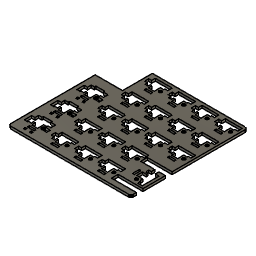
bottomplate (Autodesk Fusion 360 design; units mm, degrees)
Autodesk Fusion 360 part; units mm, degrees
(part 1 of 5)
sketch "スケッチ1" plane through (0, 0, 0) normal (0, 0, 1) x (1, 0, 0)
  line L0 (62.5173, -152.0791) -> (62.5309, -152.0926)
  line L1 (62.5309, -152.0926) -> (62.5328, -152.1022)
  line L2 (62.5328, -152.1022) -> (62.5328, -153.5905)
  line L3 (62.5328, -153.5905) -> (62.5309, -153.6001)
  line L4 (62.5309, -153.6001) -> (62.5173, -153.6136)
  line L5 (62.5173, -153.6136) -> (62.5078, -153.6155)
  line L6 (62.5078, -153.6155) -> (61.0195, -153.6155)
  line L7 (61.0195, -153.6155) -> (61.0099, -153.6136)
  line L8 (61.0099, -153.6136) -> (60.9964, -153.6001)
  line L9 (60.9964, -153.6001) -> (60.9945, -153.5905)
  line L10 (60.9945, -153.5905) -> (60.9945, -152.1022)
  line L11 (60.9945, -152.1022) -> (60.9964, -152.0926)
  line L12 (60.9964, -152.0926) -> (61.0099, -152.0791)
  line L13 (61.0099, -152.0791) -> (61.0195, -152.0772)
  line L14 (61.0195, -152.0772) -> (62.5078, -152.0772)
  line L15 (62.5078, -152.0772) -> (62.5173, -152.0791)
  line L16 (61.0445, -152.1272) -> (61.0445, -153.5655)
  line L17 (61.0445, -153.5655) -> (62.4828, -153.5655)
  line L18 (62.4828, -153.5655) -> (62.4828, -152.1272)
  line L19 (62.4828, -152.1272) -> (61.0445, -152.1272)
  line L20 (67.5775, -152.0791) -> (67.591, -152.0926)
  line L21 (67.591, -152.0926) -> (67.5929, -152.1022)
  line L22 (67.5929, -152.1022) -> (67.5929, -153.5905)
  line L23 (67.5929, -153.5905) -> (67.591, -153.6001)
  line L24 (67.591, -153.6001) -> (67.5775, -153.6136)
  line L25 (67.5775, -153.6136) -> (67.5679, -153.6155)
  line L26 (67.5679, -153.6155) -> (66.0796, -153.6155)
  line L27 (66.0796, -153.6155) -> (66.0701, -153.6136)
  line L28 (66.0701, -153.6136) -> (66.0565, -153.6001)
  line L29 (66.0565, -153.6001) -> (66.0546, -153.5905)
  line L30 (66.0546, -153.5905) -> (66.0546, -152.1022)
  line L31 (66.0546, -152.1022) -> (66.0565, -152.0926)
  line L32 (66.0565, -152.0926) -> (66.0701, -152.0791)
  line L33 (66.0701, -152.0791) -> (66.0796, -152.0772)
  line L34 (66.0796, -152.0772) -> (67.5679, -152.0772)
  line L35 (67.5679, -152.0772) -> (67.5775, -152.0791)
  line L36 (66.1046, -152.1272) -> (66.1046, -153.5655)
  line L37 (66.1046, -153.5655) -> (67.5429, -153.5655)
  line L38 (67.5429, -153.5655) -> (67.5429, -152.1272)
  line L39 (67.5429, -152.1272) -> (66.1046, -152.1272)
  line L40 (88.4346, -151.6269) -> (88.4481, -151.6404)
  line L41 (88.4481, -151.6404) -> (88.45, -151.65)
  line L42 (88.45, -151.65) -> (88.45, -153.15)
  line L43 (88.45, -153.15) -> (88.4481, -153.1596)
  line L44 (88.4481, -153.1596) -> (88.4346, -153.1731)
  line L45 (88.4346, -153.1731) -> (88.425, -153.175)
  line L46 (88.425, -153.175) -> (83.025, -153.175)
  line L47 (83.025, -153.175) -> (83.0154, -153.1731)
  line L48 (83.0154, -153.1731) -> (83.0019, -153.1596)
  line L49 (83.0019, -153.1596) -> (83, -153.15)
  line L50 (83, -153.15) -> (83, -151.65)
  line L51 (83, -151.65) -> (83.0019, -151.6404)
  line L52 (83.0019, -151.6404) -> (83.0154, -151.6269)
  line L53 (83.0154, -151.6269) -> (83.025, -151.625)
  line L54 (83.025, -151.625) -> (88.425, -151.625)
  line L55 (88.425, -151.625) -> (88.4346, -151.6269)
  line L56 (83.05, -151.675) -> (83.05, -153.125)
  line L57 (83.05, -153.125) -> (88.4, -153.125)
  line L58 (88.4, -153.125) -> (88.4, -151.675)
  line L59 (88.4, -151.675) -> (83.05, -151.675)
  line L60 (107.4846, -151.6269) -> (107.4981, -151.6404)
  line L61 (107.4981, -151.6404) -> (107.5, -151.65)
  line L62 (107.5, -151.65) -> (107.5, -153.15)
  line L63 (107.5, -153.15) -> (107.4981, -153.1596)
  line L64 (107.4981, -153.1596) -> (107.4846, -153.1731)
  line L65 (107.4846, -153.1731) -> (107.475, -153.175)
  line L66 (107.475, -153.175) -> (102.075, -153.175)
  line L67 (102.075, -153.175) -> (102.0654, -153.1731)
  line L68 (102.0654, -153.1731) -> (102.0519, -153.1596)
  line L69 (102.0519, -153.1596) -> (102.05, -153.15)
  line L70 (102.05, -153.15) -> (102.05, -151.65)
  line L71 (102.05, -151.65) -> (102.0519, -151.6404)
  line L72 (102.0519, -151.6404) -> (102.0654, -151.6269)
  line L73 (102.0654, -151.6269) -> (102.075, -151.625)
  line L74 (102.075, -151.625) -> (107.475, -151.625)
  line L75 (107.475, -151.625) -> (107.4846, -151.6269)
  line L76 (102.1, -151.675) -> (102.1, -153.125)
  line L77 (102.1, -153.125) -> (107.45, -153.125)
  line L78 (107.45, -153.125) -> (107.45, -151.675)
  line L79 (107.45, -151.675) -> (102.1, -151.675)
  line L80 (126.5346, -151.6269) -> (126.5481, -151.6404)
  line L81 (126.5481, -151.6404) -> (126.55, -151.65)
  line L82 (126.55, -151.65) -> (126.55, -153.15)
  line L83 (126.55, -153.15) -> (126.5481, -153.1596)
  line L84 (126.5481, -153.1596) -> (126.5346, -153.1731)
  line L85 (126.5346, -153.1731) -> (126.525, -153.175)
  line L86 (126.525, -153.175) -> (121.125, -153.175)
  line L87 (121.125, -153.175) -> (121.1154, -153.1731)
  line L88 (121.1154, -153.1731) -> (121.1019, -153.1596)
  line L89 (121.1019, -153.1596) -> (121.1, -153.15)
  line L90 (121.1, -153.15) -> (121.1, -151.65)
  line L91 (121.1, -151.65) -> (121.1019, -151.6404)
  line L92 (121.1019, -151.6404) -> (121.1154, -151.6269)
  line L93 (121.1154, -151.6269) -> (121.125, -151.625)
  line L94 (121.125, -151.625) -> (126.525, -151.625)
  line L95 (126.525, -151.625) -> (126.5346, -151.6269)
  line L96 (121.15, -151.675) -> (121.15, -153.125)
  line L97 (121.15, -153.125) -> (126.5, -153.125)
  line L98 (126.5, -153.125) -> (126.5, -151.675)
  line L99 (126.5, -151.675) -> (121.15, -151.675)
  line L100 (67.0033, -149.2457) -> (67.0168, -149.2592)
  line L101 (67.0168, -149.2592) -> (67.0187, -149.2687)
  line L102 (67.0187, -149.2687) -> (67.0187, -150.7687)
  line L103 (67.0187, -150.7687) -> (67.0168, -150.7783)
  line L104 (67.0168, -150.7783) -> (67.0033, -150.7918)
  line L105 (67.0033, -150.7918) -> (66.9938, -150.7937)
  line L106 (66.9938, -150.7937) -> (61.5938, -150.7937)
  line L107 (61.5938, -150.7937) -> (61.5842, -150.7918)
  line L108 (61.5842, -150.7918) -> (61.5707, -150.7783)
  line L109 (61.5707, -150.7783) -> (61.5688, -150.7687)
  line L110 (61.5688, -150.7687) -> (61.5688, -149.2687)
  line L111 (61.5688, -149.2687) -> (61.5707, -149.2592)
  line L112 (61.5707, -149.2592) -> (61.5842, -149.2457)
  line L113 (61.5842, -149.2457) -> (61.5938, -149.2438)
  line L114 (61.5938, -149.2438) -> (66.9938, -149.2438)
  line L115 (66.9938, -149.2438) -> (67.0033, -149.2457)
  line L116 (61.6188, -149.2937) -> (61.6188, -150.7438)
  line L117 (61.6188, -150.7438) -> (66.9688, -150.7438)
  line L118 (66.9688, -150.7438) -> (66.9688, -149.2937)
  line L119 (66.9688, -149.2937) -> (61.6187, -149.2937)
  line L120 (93.1758, -140.4705) -> (93.1894, -140.4841)
  line L121 (93.1894, -140.4841) -> (93.1913, -140.4936)
  line L122 (93.1913, -140.4936) -> (93.1913, -144.0655)
  line L123 (93.1913, -144.0655) -> (93.1894, -144.0751)
  line L124 (93.1894, -144.0751) -> (93.1758, -144.0886)
  line L125 (93.1758, -144.0886) -> (93.1663, -144.0905)
  line L126 (93.1663, -144.0905) -> (90.81, -144.0905)
  line L127 (90.81, -144.0905) -> (90.81, -144.9585)
  line L128 (90.81, -144.9585) -> (90.8081, -144.968)
  line L129 (90.8081, -144.968) -> (90.7946, -144.9816)
  line L130 (90.7946, -144.9816) -> (90.785, -144.9835)
  line L131 (90.785, -144.9835) -> (88.1311, -144.9835)
  line L132 (88.1311, -144.9835) -> (88.1311, -148.828)
  line L133 (88.1311, -148.828) -> (88.1311, -150.0186)
  line L134 (88.1311, -150.0186) -> (88.1292, -150.0282)
  line L135 (88.1292, -150.0282) -> (88.1157, -150.0417)
  line L136 (88.1157, -150.0417) -> (88.1061, -150.0436)
  line L137 (88.1061, -150.0436) -> (83.6413, -150.0436)
  line L138 (83.6413, -150.0436) -> (83.3436, -150.0436)
  line L139 (83.3436, -150.0436) -> (83.334, -150.0417)
  line L140 (83.334, -150.0417) -> (83.3205, -150.0282)
  line L141 (83.3205, -150.0282) -> (83.3186, -150.0186)
  line L142 (83.3186, -150.0186) -> (83.3186, -147.0671)
  line L143 (83.3186, -147.0671) -> (81.8803, -147.0671)
  line L144 (81.8803, -147.0671) -> (81.8803, -148.828)
  line L145 (81.8803, -148.828) -> (81.8784, -148.8376)
  line L146 (81.8784, -148.8376) -> (81.8649, -148.8511)
  line L147 (81.8649, -148.8511) -> (81.8553, -148.853)
  line L148 (81.8553, -148.853) -> (79.4741, -148.853)
  line L149 (79.4741, -148.853) -> (79.4645, -148.8511)
  line L150 (79.4645, -148.8511) -> (79.451, -148.8376)
  line L151 (79.451, -148.8376) -> (79.4491, -148.828)
  line L152 (79.4491, -148.828) -> (79.4491, -146.7694)
  line L153 (79.4491, -146.7694) -> (77.0928, -146.7694)
  line L154 (77.0928, -146.7694) -> (77.0833, -146.7675)
  line L155 (77.0833, -146.7675) -> (77.0697, -146.754)
  line L156 (77.0697, -146.754) -> (77.0678, -146.7444)
  line L157 (77.0678, -146.7444) -> (77.0678, -143.4702)
  line L158 (77.0678, -143.4702) -> (77.0697, -143.4606)
  line L159 (77.0697, -143.4606) -> (77.0833, -143.4471)
  line L160 (77.0833, -143.4471) -> (77.0928, -143.4452)
  line L161 (77.0928, -143.4452) -> (79.4491, -143.4452)
  line L162 (79.4491, -143.4452) -> (79.4491, -140.4936)
  line L163 (79.4491, -140.4936) -> (79.451, -140.4841)
  line L164 (79.451, -140.4841) -> (79.4645, -140.4705)
  line L165 (79.4645, -140.4705) -> (79.4741, -140.4686)
  line L166 (79.4741, -140.4686) -> (93.1663, -140.4686)
  line L167 (93.1663, -140.4686) -> (93.1758, -140.4705)
  line L168 (79.4991, -140.5186) -> (79.4991, -143.4702)
  line L169 (79.4991, -143.4702) -> (79.4972, -143.4798)
  line L170 (79.4972, -143.4798) -> (79.4836, -143.4933)
  line L171 (79.4836, -143.4933) -> (79.4741, -143.4952)
  line L172 (79.4741, -143.4952) -> (77.1178, -143.4952)
  line L173 (77.1178, -143.4952) -> (77.1178, -146.7194)
  line L174 (77.1178, -146.7194) -> (79.4741, -146.7194)
  line L175 (79.4741, -146.7194) -> (79.4836, -146.7213)
  line L176 (79.4836, -146.7213) -> (79.4972, -146.7348)
  line L177 (79.4972, -146.7348) -> (79.4991, -146.7444)
  line L178 (79.4991, -146.7444) -> (79.4991, -148.803)
  line L179 (79.4991, -148.803) -> (81.8303, -148.803)
  line L180 (81.8303, -148.803) -> (81.8303, -147.0421)
  line L181 (81.8303, -147.0421) -> (81.8322, -147.0325)
  line L182 (81.8322, -147.0325) -> (81.8458, -147.019)
  line L183 (81.8458, -147.019) -> (81.8553, -147.0171)
  line L184 (81.8553, -147.0171) -> (83.3436, -147.0171)
  line L185 (83.3436, -147.0171) -> (83.3532, -147.019)
  line L186 (83.3532, -147.019) -> (83.3667, -147.0325)
  line L187 (83.3667, -147.0325) -> (83.3686, -147.0421)
  line L188 (83.3686, -147.0421) -> (83.3686, -149.9936)
  line L189 (83.3686, -149.9936) -> (83.6413, -149.9936)
  line L190 (83.6413, -149.9936) -> (88.0811, -149.9936)
  line L191 (88.0811, -149.9936) -> (88.0811, -148.828)
  line L192 (88.0811, -148.828) -> (88.0811, -144.9585)
  line L193 (88.0811, -144.9585) -> (88.083, -144.9489)
  line L194 (88.083, -144.9489) -> (88.0965, -144.9354)
  line L195 (88.0965, -144.9354) -> (88.1061, -144.9335)
  line L196 (88.1061, -144.9335) -> (90.76, -144.9335)
  line L197 (90.76, -144.9335) -> (90.76, -144.0655)
  line L198 (90.76, -144.0655) -> (90.7619, -144.0559)
  line L199 (90.7619, -144.0559) -> (90.7754, -144.0424)
  line L200 (90.7754, -144.0424) -> (90.785, -144.0405)
  line L201 (90.785, -144.0405) -> (93.1413, -144.0405)
  line L202 (93.1413, -144.0405) -> (93.1413, -140.5186)
  line L203 (93.1413, -140.5186) -> (79.4991, -140.5186)
  line L204 (112.2258, -140.4705) -> (112.2394, -140.4841)
  line L205 (112.2394, -140.4841) -> (112.2413, -140.4936)
  line L206 (112.2413, -140.4936) -> (112.2413, -144.0655)
  line L207 (112.2413, -144.0655) -> (112.2394, -144.0751)
  line L208 (112.2394, -144.0751) -> (112.2258, -144.0886)
  line L209 (112.2258, -144.0886) -> (112.2163, -144.0905)
  line L210 (112.2163, -144.0905) -> (109.86, -144.0905)
  line L211 (109.86, -144.0905) -> (109.86, -144.9585)
  line L212 (109.86, -144.9585) -> (109.8581, -144.968)
  line L213 (109.8581, -144.968) -> (109.8446, -144.9816)
  line L214 (109.8446, -144.9816) -> (109.835, -144.9835)
  line L215 (109.835, -144.9835) -> (107.1811, -144.9835)
  line L216 (107.1811, -144.9835) -> (107.1811, -148.828)
  line L217 (107.1811, -148.828) -> (107.1811, -150.0186)
  line L218 (107.1811, -150.0186) -> (107.1792, -150.0282)
  line L219 (107.1792, -150.0282) -> (107.1657, -150.0417)
  line L220 (107.1657, -150.0417) -> (107.1561, -150.0436)
  line L221 (107.1561, -150.0436) -> (102.6913, -150.0436)
  line L222 (102.6913, -150.0436) -> (102.3936, -150.0436)
  line L223 (102.3936, -150.0436) -> (102.384, -150.0417)
  line L224 (102.384, -150.0417) -> (102.3705, -150.0282)
  line L225 (102.3705, -150.0282) -> (102.3686, -150.0186)
  line L226 (102.3686, -150.0186) -> (102.3686, -147.0671)
  line L227 (102.3686, -147.0671) -> (100.9303, -147.0671)
  line L228 (100.9303, -147.0671) -> (100.9303, -148.828)
  line L229 (100.9303, -148.828) -> (100.9284, -148.8376)
  line L230 (100.9284, -148.8376) -> (100.9149, -148.8511)
  line L231 (100.9149, -148.8511) -> (100.9053, -148.853)
  line L232 (100.9053, -148.853) -> (98.5241, -148.853)
  line L233 (98.5241, -148.853) -> (98.5145, -148.8511)
  line L234 (98.5145, -148.8511) -> (98.501, -148.8376)
  line L235 (98.501, -148.8376) -> (98.4991, -148.828)
  line L236 (98.4991, -148.828) -> (98.4991, -146.7694)
  line L237 (98.4991, -146.7694) -> (96.1428, -146.7694)
  line L238 (96.1428, -146.7694) -> (96.1333, -146.7675)
  line L239 (96.1333, -146.7675) -> (96.1197, -146.754)
  line L240 (96.1197, -146.754) -> (96.1178, -146.7444)
  line L241 (96.1178, -146.7444) -> (96.1178, -143.4702)
  line L242 (96.1178, -143.4702) -> (96.1197, -143.4606)
  line L243 (96.1197, -143.4606) -> (96.1333, -143.4471)
  line L244 (96.1333, -143.4471) -> (96.1428, -143.4452)
  line L245 (96.1428, -143.4452) -> (98.4991, -143.4452)
  line L246 (98.4991, -143.4452) -> (98.4991, -140.4936)
  line L247 (98.4991, -140.4936) -> (98.501, -140.4841)
  line L248 (98.501, -140.4841) -> (98.5145, -140.4705)
  line L249 (98.5145, -140.4705) -> (98.5241, -140.4686)
  line L250 (98.5241, -140.4686) -> (112.2163, -140.4686)
  line L251 (112.2163, -140.4686) -> (112.2258, -140.4705)
  line L252 (98.5491, -140.5186) -> (98.5491, -143.4702)
  line L253 (98.5491, -143.4702) -> (98.5472, -143.4798)
  line L254 (98.5472, -143.4798) -> (98.5336, -143.4933)
  line L255 (98.5336, -143.4933) -> (98.5241, -143.4952)
  line L256 (98.5241, -143.4952) -> (96.1678, -143.4952)
  line L257 (96.1678, -143.4952) -> (96.1678, -146.7194)
  line L258 (96.1678, -146.7194) -> (98.5241, -146.7194)
  line L259 (98.5241, -146.7194) -> (98.5336, -146.7213)
  line L260 (98.5336, -146.7213) -> (98.5472, -146.7348)
  line L261 (98.5472, -146.7348) -> (98.5491, -146.7444)
  line L262 (98.5491, -146.7444) -> (98.5491, -148.803)
  line L263 (98.5491, -148.803) -> (100.8803, -148.803)
  line L264 (100.8803, -148.803) -> (100.8803, -147.0421)
  line L265 (100.8803, -147.0421) -> (100.8822, -147.0325)
  line L266 (100.8822, -147.0325) -> (100.8958, -147.019)
  line L267 (100.8958, -147.019) -> (100.9053, -147.0171)
  line L268 (100.9053, -147.0171) -> (102.3936, -147.0171)
  line L269 (102.3936, -147.0171) -> (102.4032, -147.019)
  line L270 (102.4032, -147.019) -> (102.4167, -147.0325)
  line L271 (102.4167, -147.0325) -> (102.4186, -147.0421)
  line L272 (102.4186, -147.0421) -> (102.4186, -149.9936)
  line L273 (102.4186, -149.9936) -> (102.6913, -149.9936)
  line L274 (102.6913, -149.9936) -> (107.1311, -149.9936)
  line L275 (107.1311, -149.9936) -> (107.1311, -148.828)
  line L276 (107.1311, -148.828) -> (107.1311, -144.9585)
  line L277 (107.1311, -144.9585) -> (107.133, -144.9489)
  line L278 (107.133, -144.9489) -> (107.1465, -144.9354)
  line L279 (107.1465, -144.9354) -> (107.1561, -144.9335)
  line L280 (107.1561, -144.9335) -> (109.81, -144.9335)
  line L281 (109.81, -144.9335) -> (109.81, -144.0655)
  line L282 (109.81, -144.0655) -> (109.8119, -144.0559)
  line L283 (109.8119, -144.0559) -> (109.8254, -144.0424)
  line L284 (109.8254, -144.0424) -> (109.835, -144.0405)
  line L285 (109.835, -144.0405) -> (112.1913, -144.0405)
  line L286 (112.1913, -144.0405) -> (112.1913, -140.5186)
  line L287 (112.1913, -140.5186) -> (98.5491, -140.5186)
  line L288 (131.2758, -140.4705) -> (131.2894, -140.4841)
  line L289 (131.2894, -140.4841) -> (131.2913, -140.4936)
  line L290 (131.2913, -140.4936) -> (131.2913, -144.0655)
  line L291 (131.2913, -144.0655) -> (131.2894, -144.0751)
  line L292 (131.2894, -144.0751) -> (131.2758, -144.0886)
  line L293 (131.2758, -144.0886) -> (131.2663, -144.0905)
  line L294 (131.2663, -144.0905) -> (128.91, -144.0905)
  line L295 (128.91, -144.0905) -> (128.91, -144.9585)
  line L296 (128.91, -144.9585) -> (128.9081, -144.968)
  line L297 (128.9081, -144.968) -> (128.8946, -144.9816)
  line L298 (128.8946, -144.9816) -> (128.885, -144.9835)
  line L299 (128.885, -144.9835) -> (126.2311, -144.9835)
  line L300 (126.2311, -144.9835) -> (126.2311, -148.828)
  line L301 (126.2311, -148.828) -> (126.2311, -150.0186)
  line L302 (126.2311, -150.0186) -> (126.2292, -150.0282)
  line L303 (126.2292, -150.0282) -> (126.2157, -150.0417)
  line L304 (126.2157, -150.0417) -> (126.2061, -150.0436)
  line L305 (126.2061, -150.0436) -> (121.7413, -150.0436)
  line L306 (121.7413, -150.0436) -> (121.4436, -150.0436)
  line L307 (121.4436, -150.0436) -> (121.434, -150.0417)
  line L308 (121.434, -150.0417) -> (121.4205, -150.0282)
  line L309 (121.4205, -150.0282) -> (121.4186, -150.0186)
  line L310 (121.4186, -150.0186) -> (121.4186, -147.0671)
  line L311 (121.4186, -147.0671) -> (119.9803, -147.0671)
  line L312 (119.9803, -147.0671) -> (119.9803, -148.828)
  line L313 (119.9803, -148.828) -> (119.9784, -148.8376)
  line L314 (119.9784, -148.8376) -> (119.9649, -148.8511)
  line L315 (119.9649, -148.8511) -> (119.9553, -148.853)
  line L316 (119.9553, -148.853) -> (117.5741, -148.853)
  line L317 (117.5741, -148.853) -> (117.5645, -148.8511)
  line L318 (117.5645, -148.8511) -> (117.551, -148.8376)
  line L319 (117.551, -148.8376) -> (117.5491, -148.828)
  line L320 (117.5491, -148.828) -> (117.5491, -146.7694)
  line L321 (117.5491, -146.7694) -> (115.1928, -146.7694)
  line L322 (115.1928, -146.7694) -> (115.1833, -146.7675)
  line L323 (115.1833, -146.7675) -> (115.1697, -146.754)
  line L324 (115.1697, -146.754) -> (115.1678, -146.7444)
  line L325 (115.1678, -146.7444) -> (115.1678, -143.4702)
  line L326 (115.1678, -143.4702) -> (115.1697, -143.4606)
  line L327 (115.1697, -143.4606) -> (115.1833, -143.4471)
  line L328 (115.1833, -143.4471) -> (115.1928, -143.4452)
  line L329 (115.1928, -143.4452) -> (117.5491, -143.4452)
  line L330 (117.5491, -143.4452) -> (117.5491, -140.4936)
  line L331 (117.5491, -140.4936) -> (117.551, -140.4841)
  line L332 (117.551, -140.4841) -> (117.5645, -140.4705)
  line L333 (117.5645, -140.4705) -> (117.5741, -140.4686)
  line L334 (117.5741, -140.4686) -> (131.2663, -140.4686)
  line L335 (131.2663, -140.4686) -> (131.2758, -140.4705)
  line L336 (117.5991, -140.5186) -> (117.5991, -143.4702)
  line L337 (117.5991, -143.4702) -> (117.5972, -143.4798)
  line L338 (117.5972, -143.4798) -> (117.5836, -143.4933)
  line L339 (117.5836, -143.4933) -> (117.5741, -143.4952)
  line L340 (117.5741, -143.4952) -> (115.2178, -143.4952)
  line L341 (115.2178, -143.4952) -> (115.2178, -146.7194)
  line L342 (115.2178, -146.7194) -> (117.5741, -146.7194)
  line L343 (117.5741, -146.7194) -> (117.5836, -146.7213)
  line L344 (117.5836, -146.7213) -> (117.5972, -146.7348)
  line L345 (117.5972, -146.7348) -> (117.5991, -146.7444)
  line L346 (117.5991, -146.7444) -> (117.5991, -148.803)
  line L347 (117.5991, -148.803) -> (119.9303, -148.803)
  line L348 (119.9303, -148.803) -> (119.9303, -147.0421)
  line L349 (119.9303, -147.0421) -> (119.9322, -147.0325)
  line L350 (119.9322, -147.0325) -> (119.9458, -147.019)
  line L351 (119.9458, -147.019) -> (119.9553, -147.0171)
  line L352 (119.9553, -147.0171) -> (121.4436, -147.0171)
  line L353 (121.4436, -147.0171) -> (121.4532, -147.019)
  line L354 (121.4532, -147.019) -> (121.4667, -147.0325)
  line L355 (121.4667, -147.0325) -> (121.4686, -147.0421)
  line L356 (121.4686, -147.0421) -> (121.4686, -149.9936)
  line L357 (121.4686, -149.9936) -> (121.7413, -149.9936)
  line L358 (121.7413, -149.9936) -> (126.1811, -149.9936)
  line L359 (126.1811, -149.9936) -> (126.1811, -148.828)
  line L360 (126.1811, -148.828) -> (126.1811, -144.9585)
  line L361 (126.1811, -144.9585) -> (126.183, -144.9489)
  line L362 (126.183, -144.9489) -> (126.1965, -144.9354)
  line L363 (126.1965, -144.9354) -> (126.2061, -144.9335)
  line L364 (126.2061, -144.9335) -> (128.86, -144.9335)
  line L365 (128.86, -144.9335) -> (128.86, -144.0655)
  line L366 (128.86, -144.0655) -> (128.8619, -144.0559)
  line L367 (128.8619, -144.0559) -> (128.8754, -144.0424)
  line L368 (128.8754, -144.0424) -> (128.885, -144.0405)
  line L369 (128.885, -144.0405) -> (131.2413, -144.0405)
  line L370 (131.2413, -144.0405) -> (131.2413, -140.5186)
  line L371 (131.2413, -140.5186) -> (117.5991, -140.5186)
  line L372 (90.9961, -146.4402) -> (91.2008, -146.4951)
  line L373 (91.2008, -146.4951) -> (91.3928, -146.5846)
  line L374 (91.3928, -146.5846) -> (91.5664, -146.7062)
  line L375 (91.5664, -146.7062) -> (91.7162, -146.856)
  line L376 (91.7162, -146.856) -> (91.8378, -147.0296)
  line L377 (91.8378, -147.0296) -> (91.9273, -147.2216)
  line L378 (91.9273, -147.2216) -> (91.9822, -147.4263)
  line L379 (91.9822, -147.4263) -> (92.0006, -147.6374)
  line L380 (92.0006, -147.6374) -> (91.9822, -147.8485)
  line L381 (91.9822, -147.8485) -> (91.9273, -148.0531)
  line L382 (91.9273, -148.0531) -> (91.8378, -148.2452)
  line L383 (91.8378, -148.2452) -> (91.7162, -148.4188)
  line L384 (91.7162, -148.4188) -> (91.5664, -148.5686)
  line L385 (91.5664, -148.5686) -> (91.3928, -148.6901)
  line L386 (91.3928, -148.6901) -> (91.2008, -148.7797)
  line L387 (91.2008, -148.7797) -> (90.9961, -148.8345)
  line L388 (90.9961, -148.8345) -> (90.785, -148.853)
  line L389 (90.785, -148.853) -> (90.5739, -148.8345)
  line L390 (90.5739, -148.8345) -> (90.3692, -148.7797)
  line L391 (90.3692, -148.7797) -> (90.1772, -148.6901)
  line L392 (90.1772, -148.6901) -> (90.0036, -148.5686)
  line L393 (90.0036, -148.5686) -> (89.8538, -148.4188)
  line L394 (89.8538, -148.4188) -> (89.7322, -148.2452)
  line L395 (89.7322, -148.2452) -> (89.6427, -148.0531)
  line L396 (89.6427, -148.0531) -> (89.5879, -147.8485)
  line L397 (89.5879, -147.8485) -> (89.5694, -147.6374)
  line L398 (89.5694, -147.6374) -> (89.5879, -147.4263)
  line L399 (89.5879, -147.4263) -> (89.6427, -147.2216)
  line L400 (89.6427, -147.2216) -> (89.7322, -147.0296)
  line L401 (89.7322, -147.0296) -> (89.8538, -146.856)
  line L402 (89.8538, -146.856) -> (90.0036, -146.7062)
  line L403 (90.0036, -146.7062) -> (90.1772, -146.5846)
  line L404 (90.1772, -146.5846) -> (90.3692, -146.4951)
  line L405 (90.3692, -146.4951) -> (90.5739, -146.4402)
  line L406 (90.5739, -146.4402) -> (90.785, -146.4218)
  line L407 (90.785, -146.4218) -> (90.9961, -146.4402)
  line L408 (89.6343, -147.8525) -> (89.6934, -148.0603)
  line L409 (89.6934, -148.0603) -> (89.7897, -148.2536)
  line L410 (89.7897, -148.2536) -> (89.9199, -148.426)
  line L411 (89.9199, -148.426) -> (90.0796, -148.5715)
  line L412 (90.0796, -148.5715) -> (90.2632, -148.6853)
  line L413 (90.2632, -148.6853) -> (90.4647, -148.7633)
  line L414 (90.4647, -148.7633) -> (90.677, -148.803)
  line L415 (90.677, -148.803) -> (90.893, -148.803)
  line L416 (90.893, -148.803) -> (91.1054, -148.7633)
  line L417 (91.1054, -148.7633) -> (91.3068, -148.6853)
  line L418 (91.3068, -148.6853) -> (91.4905, -148.5715)
  line L419 (91.4905, -148.5715) -> (91.6501, -148.426)
  line L420 (91.6501, -148.426) -> (91.7803, -148.2536)
  line L421 (91.7803, -148.2536) -> (91.8766, -148.0603)
  line L422 (91.8766, -148.0603) -> (91.9357, -147.8525)
  line L423 (91.9357, -147.8525) -> (91.9556, -147.6374)
  line L424 (91.9556, -147.6374) -> (91.9357, -147.4223)
  line L425 (91.9357, -147.4223) -> (91.8766, -147.2145)
  line L426 (91.8766, -147.2145) -> (91.7803, -147.0211)
  line L427 (91.7803, -147.0211) -> (91.6501, -146.8487)
  line L428 (91.6501, -146.8487) -> (91.4905, -146.7032)
  line L429 (91.4905, -146.7032) -> (91.3068, -146.5895)
  line L430 (91.3068, -146.5895) -> (91.1054, -146.5114)
  line L431 (91.1054, -146.5114) -> (90.893, -146.4718)
  line L432 (90.893, -146.4718) -> (90.677, -146.4718)
  line L433 (90.677, -146.4718) -> (90.4647, -146.5114)
  line L434 (90.4647, -146.5114) -> (90.2632, -146.5895)
  line L435 (90.2632, -146.5895) -> (90.0796, -146.7032)
  line L436 (90.0796, -146.7032) -> (89.9199, -146.8487)
  line L437 (89.9199, -146.8487) -> (89.7897, -147.0211)
  line L438 (89.7897, -147.0211) -> (89.6934, -147.2145)
  line L439 (89.6934, -147.2145) -> (89.6343, -147.4223)
  line L440 (89.6343, -147.4223) -> (89.6144, -147.6374)
  line L441 (89.6144, -147.6374) -> (89.6343, -147.8525)
  line L442 (110.0461, -146.4402) -> (110.2508, -146.4951)
  line L443 (110.2508, -146.4951) -> (110.4428, -146.5846)
  line L444 (110.4428, -146.5846) -> (110.6164, -146.7062)
  line L445 (110.6164, -146.7062) -> (110.7662, -146.856)
  line L446 (110.7662, -146.856) -> (110.8878, -147.0296)
  line L447 (110.8878, -147.0296) -> (110.9773, -147.2216)
  line L448 (110.9773, -147.2216) -> (111.0322, -147.4263)
  line L449 (111.0322, -147.4263) -> (111.0506, -147.6374)
  line L450 (111.0506, -147.6374) -> (111.0322, -147.8485)
  line L451 (111.0322, -147.8485) -> (110.9773, -148.0531)
  line L452 (110.9773, -148.0531) -> (110.8878, -148.2452)
  line L453 (110.8878, -148.2452) -> (110.7662, -148.4188)
  line L454 (110.7662, -148.4188) -> (110.6164, -148.5686)
  line L455 (110.6164, -148.5686) -> (110.4428, -148.6901)
  line L456 (110.4428, -148.6901) -> (110.2508, -148.7797)
  line L457 (110.2508, -148.7797) -> (110.0461, -148.8345)
  line L458 (110.0461, -148.8345) -> (109.835, -148.853)
  line L459 (109.835, -148.853) -> (109.6239, -148.8345)
  line L460 (109.6239, -148.8345) -> (109.4192, -148.7797)
  line L461 (109.4192, -148.7797) -> (109.2272, -148.6901)
  line L462 (109.2272, -148.6901) -> (109.0536, -148.5686)
  line L463 (109.0536, -148.5686) -> (108.9038, -148.4188)
  line L464 (108.9038, -148.4188) -> (108.7822, -148.2452)
  line L465 (108.7822, -148.2452) -> (108.6927, -148.0531)
  line L466 (108.6927, -148.0531) -> (108.6379, -147.8485)
  line L467 (108.6379, -147.8485) -> (108.6194, -147.6374)
  line L468 (108.6194, -147.6374) -> (108.6379, -147.4263)
  line L469 (108.6379, -147.4263) -> (108.6927, -147.2216)
  line L470 (108.6927, -147.2216) -> (108.7822, -147.0296)
  line L471 (108.7822, -147.0296) -> (108.9038, -146.856)
  line L472 (108.9038, -146.856) -> (109.0536, -146.7062)
  line L473 (109.0536, -146.7062) -> (109.2272, -146.5846)
  line L474 (109.2272, -146.5846) -> (109.4192, -146.4951)
  line L475 (109.4192, -146.4951) -> (109.6239, -146.4402)
  line L476 (109.6239, -146.4402) -> (109.835, -146.4218)
  line L477 (109.835, -146.4218) -> (110.0461, -146.4402)
  line L478 (108.6843, -147.8525) -> (108.7434, -148.0603)
  line L479 (108.7434, -148.0603) -> (108.8397, -148.2536)
  line L480 (108.8397, -148.2536) -> (108.9699, -148.426)
  line L481 (108.9699, -148.426) -> (109.1296, -148.5715)
  line L482 (109.1296, -148.5715) -> (109.3132, -148.6853)
  line L483 (109.3132, -148.6853) -> (109.5147, -148.7633)
  line L484 (109.5147, -148.7633) -> (109.727, -148.803)
  line L485 (109.727, -148.803) -> (109.943, -148.803)
  line L486 (109.943, -148.803) -> (110.1554, -148.7633)
  line L487 (110.1554, -148.7633) -> (110.3568, -148.6853)
  line L488 (110.3568, -148.6853) -> (110.5405, -148.5715)
  line L489 (110.5405, -148.5715) -> (110.7001, -148.426)
  line L490 (110.7001, -148.426) -> (110.8303, -148.2536)
  line L491 (110.8303, -148.2536) -> (110.9266, -148.0603)
  line L492 (110.9266, -148.0603) -> (110.9857, -147.8525)
  line L493 (110.9857, -147.8525) -> (111.0056, -147.6374)
  line L494 (111.0056, -147.6374) -> (110.9857, -147.4223)
  line L495 (110.9857, -147.4223) -> (110.9266, -147.2145)
  line L496 (110.9266, -147.2145) -> (110.8303, -147.0211)
  line L497 (110.8303, -147.0211) -> (110.7001, -146.8487)
  line L498 (110.7001, -146.8487) -> (110.5405, -146.7032)
  line L499 (110.5405, -146.7032) -> (110.3568, -146.5895)
  line L500 (110.3568, -146.5895) -> (110.1554, -146.5114)
  line L501 (110.1554, -146.5114) -> (109.943, -146.4718)
  line L502 (109.943, -146.4718) -> (109.727, -146.4718)
  line L503 (109.727, -146.4718) -> (109.5147, -146.5114)
  line L504 (109.5147, -146.5114) -> (109.3132, -146.5895)
  line L505 (109.3132, -146.5895) -> (109.1296, -146.7032)
  line L506 (109.1296, -146.7032) -> (108.9699, -146.8487)
  line L507 (108.9699, -146.8487) -> (108.8397, -147.0211)
  line L508 (108.8397, -147.0211) -> (108.7434, -147.2145)
  line L509 (108.7434, -147.2145) -> (108.6843, -147.4223)
  line L510 (108.6843, -147.4223) -> (108.6644, -147.6374)
  line L511 (108.6644, -147.6374) -> (108.6843, -147.8525)
  line L512 (129.0961, -146.4402) -> (129.3008, -146.4951)
  line L513 (129.3008, -146.4951) -> (129.4928, -146.5846)
  line L514 (129.4928, -146.5846) -> (129.6664, -146.7062)
  line L515 (129.6664, -146.7062) -> (129.8162, -146.856)
  line L516 (129.8162, -146.856) -> (129.9378, -147.0296)
  line L517 (129.9378, -147.0296) -> (130.0273, -147.2216)
  line L518 (130.0273, -147.2216) -> (130.0822, -147.4263)
  line L519 (130.0822, -147.4263) -> (130.1006, -147.6374)
  line L520 (130.1006, -147.6374) -> (130.0822, -147.8485)
  line L521 (130.0822, -147.8485) -> (130.0273, -148.0531)
  line L522 (130.0273, -148.0531) -> (129.9378, -148.2452)
  line L523 (129.9378, -148.2452) -> (129.8162, -148.4188)
  line L524 (129.8162, -148.4188) -> (129.6664, -148.5686)
  line L525 (129.6664, -148.5686) -> (129.4928, -148.6901)
  line L526 (129.4928, -148.6901) -> (129.3008, -148.7797)
  line L527 (129.3008, -148.7797) -> (129.0961, -148.8345)
  line L528 (129.0961, -148.8345) -> (128.885, -148.853)
  line L529 (128.885, -148.853) -> (128.6739, -148.8345)
  line L530 (128.6739, -148.8345) -> (128.4692, -148.7797)
  line L531 (128.4692, -148.7797) -> (128.2772, -148.6901)
  line L532 (128.2772, -148.6901) -> (128.1036, -148.5686)
  line L533 (128.1036, -148.5686) -> (127.9538, -148.4188)
  line L534 (127.9538, -148.4188) -> (127.8322, -148.2452)
  line L535 (127.8322, -148.2452) -> (127.7427, -148.0531)
  line L536 (127.7427, -148.0531) -> (127.6879, -147.8485)
  line L537 (127.6879, -147.8485) -> (127.6694, -147.6374)
  line L538 (127.6694, -147.6374) -> (127.6879, -147.4263)
  line L539 (127.6879, -147.4263) -> (127.7427, -147.2216)
  line L540 (127.7427, -147.2216) -> (127.8322, -147.0296)
  line L541 (127.8322, -147.0296) -> (127.9538, -146.856)
  line L542 (127.9538, -146.856) -> (128.1036, -146.7062)
  line L543 (128.1036, -146.7062) -> (128.2772, -146.5846)
  line L544 (128.2772, -146.5846) -> (128.4692, -146.4951)
  line L545 (128.4692, -146.4951) -> (128.6739, -146.4402)
  line L546 (128.6739, -146.4402) -> (128.885, -146.4218)
  line L547 (128.885, -146.4218) -> (129.0961, -146.4402)
  line L548 (127.7343, -147.8525) -> (127.7934, -148.0603)
  line L549 (127.7934, -148.0603) -> (127.8897, -148.2536)
  line L550 (127.8897, -148.2536) -> (128.0199, -148.426)
  line L551 (128.0199, -148.426) -> (128.1796, -148.5715)
  line L552 (128.1796, -148.5715) -> (128.3632, -148.6853)
  line L553 (128.3632, -148.6853) -> (128.5647, -148.7633)
  line L554 (128.5647, -148.7633) -> (128.777, -148.803)
  line L555 (128.777, -148.803) -> (128.993, -148.803)
  line L556 (128.993, -148.803) -> (129.2054, -148.7633)
  line L557 (129.2054, -148.7633) -> (129.4068, -148.6853)
  line L558 (129.4068, -148.6853) -> (129.5905, -148.5715)
  line L559 (129.5905, -148.5715) -> (129.7501, -148.426)
  line L560 (129.7501, -148.426) -> (129.8803, -148.2536)
  line L561 (129.8803, -148.2536) -> (129.9766, -148.0603)
  line L562 (129.9766, -148.0603) -> (130.0357, -147.8525)
  line L563 (130.0357, -147.8525) -> (130.0556, -147.6374)
  line L564 (130.0556, -147.6374) -> (130.0357, -147.4223)
  line L565 (130.0357, -147.4223) -> (129.9766, -147.2145)
  line L566 (129.9766, -147.2145) -> (129.8803, -147.0211)
  line L567 (129.8803, -147.0211) -> (129.7501, -146.8487)
  line L568 (129.7501, -146.8487) -> (129.5905, -146.7032)
  line L569 (129.5905, -146.7032) -> (129.4068, -146.5895)
  line L570 (129.4068, -146.5895) -> (129.2054, -146.5114)
  line L571 (129.2054, -146.5114) -> (128.993, -146.4718)
  line L572 (128.993, -146.4718) -> (128.777, -146.4718)
  line L573 (128.777, -146.4718) -> (128.5647, -146.5114)
  line L574 (128.5647, -146.5114) -> (128.3632, -146.5895)
  line L575 (128.3632, -146.5895) -> (128.1796, -146.7032)
  line L576 (128.1796, -146.7032) -> (128.0199, -146.8487)
  line L577 (128.0199, -146.8487) -> (127.8897, -147.0211)
  line L578 (127.8897, -147.0211) -> (127.7934, -147.2145)
  line L579 (127.7934, -147.2145) -> (127.7343, -147.4223)
  line L580 (127.7343, -147.4223) -> (127.7144, -147.6374)
  line L581 (127.7144, -147.6374) -> (127.7343, -147.8525)
  line L582 (67.8751, -136.8987) -> (67.8887, -136.9122)
  line L583 (67.8887, -136.9122) -> (67.8906, -136.9218)
  line L584 (67.8906, -136.9218) -> (67.8906, -138.0874)
  line L585 (67.8906, -138.0874) -> (71.735, -138.0874)
  line L586 (71.735, -138.0874) -> (71.7446, -138.0893)
  line L587 (71.7446, -138.0893) -> (71.7581, -138.1028)
  line L588 (71.7581, -138.1028) -> (71.76, -138.1124)
  line L589 (71.76, -138.1124) -> (71.76, -141.6843)
  line L590 (71.76, -141.6843) -> (71.7581, -141.6938)
  line L591 (71.7581, -141.6938) -> (71.7446, -141.7074)
  line L592 (71.7446, -141.7074) -> (71.735, -141.7093)
  line L593 (71.735, -141.7093) -> (69.3788, -141.7093)
  line L594 (69.3788, -141.7093) -> (69.3788, -142.5772)
  line L595 (69.3788, -142.5772) -> (69.3769, -142.5868)
  line L596 (69.3769, -142.5868) -> (69.3633, -142.6003)
  line L597 (69.3633, -142.6003) -> (69.3538, -142.6022)
  line L598 (69.3538, -142.6022) -> (66.6999, -142.6022)
  line L599 (66.6999, -142.6022) -> (66.6999, -146.4467)
  line L600 (66.6999, -146.4468) -> (66.6999, -147.6374)
  line L601 (66.6999, -147.6374) -> (66.698, -147.6469)
  line L602 (66.698, -147.6469) -> (66.6844, -147.6605)
  line L603 (66.6844, -147.6605) -> (66.6749, -147.6624)
  line L604 (66.6749, -147.6624) -> (62.21, -147.6624)
  line L605 (62.21, -147.6624) -> (61.9124, -147.6624)
  line L606 (61.9124, -147.6624) -> (61.9028, -147.6605)
  line L607 (61.9028, -147.6605) -> (61.8893, -147.6469)
  line L608 (61.8893, -147.6469) -> (61.8874, -147.6374)
  line L609 (61.8874, -147.6374) -> (61.8874, -144.6858)
  line L610 (61.8874, -144.6858) -> (60.4491, -144.6858)
  line L611 (60.4491, -144.6858) -> (60.4491, -146.4467)
  line L612 (60.4491, -146.4468) -> (60.4472, -146.4563)
  line L613 (60.4472, -146.4563) -> (60.4336, -146.4698)
  line L614 (60.4336, -146.4698) -> (60.4241, -146.4717)
  line L615 (60.4241, -146.4717) -> (58.0678, -146.4717)
  line L616 (58.0678, -146.4717) -> (58.0678, -147.0421)
  line L617 (58.0678, -147.0421) -> (58.0659, -147.0516)
  line L618 (58.0659, -147.0516) -> (58.0524, -147.0652)
  line L619 (58.0524, -147.0652) -> (58.0428, -147.0671)
  line L620 (58.0428, -147.0671) -> (55.364, -147.0671)
  line L621 (55.364, -147.0671) -> (55.3544, -147.0652)
  line L622 (55.3544, -147.0652) -> (55.3409, -147.0516)
  line L623 (55.3409, -147.0516) -> (55.339, -147.0421)
  line L624 (55.339, -147.0421) -> (55.339, -141.0889)
  line L625 (55.339, -141.0889) -> (55.3409, -141.0794)
  line L626 (55.3409, -141.0794) -> (55.3544, -141.0658)
  line L627 (55.3544, -141.0658) -> (55.364, -141.0639)
  line L628 (55.364, -141.0639) -> (58.0178, -141.0639)
  line L629 (58.0178, -141.0639) -> (58.0178, -138.1124)
  line L630 (58.0178, -138.1124) -> (58.0197, -138.1028)
  line L631 (58.0197, -138.1028) -> (58.0333, -138.0893)
  line L632 (58.0333, -138.0893) -> (58.0428, -138.0874)
  line L633 (58.0428, -138.0874) -> (60.6968, -138.0874)
  line L634 (60.6968, -138.0874) -> (60.6968, -136.9218)
  line L635 (60.6968, -136.9218) -> (60.6987, -136.9122)
  line L636 (60.6987, -136.9122) -> (60.7123, -136.8987)
  line L637 (60.7123, -136.8987) -> (60.7218, -136.8968)
  line L638 (60.7218, -136.8968) -> (67.8656, -136.8968)
  line L639 (67.8656, -136.8968) -> (67.8751, -136.8987)
  line L640 (60.7468, -136.9468) -> (60.7468, -138.1124)
  line L641 (60.7468, -138.1124) -> (60.7449, -138.1219)
  line L642 (60.7449, -138.1219) -> (60.7314, -138.1355)
  line L643 (60.7314, -138.1355) -> (60.7218, -138.1374)
  line L644 (60.7218, -138.1374) -> (58.0678, -138.1374)
  line L645 (58.0678, -138.1374) -> (58.0678, -141.0889)
  line L646 (58.0678, -141.0889) -> (58.0659, -141.0985)
  line L647 (58.0659, -141.0985) -> (58.0524, -141.112)
  line L648 (58.0524, -141.112) -> (58.0428, -141.1139)
  line L649 (58.0428, -141.1139) -> (55.389, -141.1139)
  line L650 (55.389, -141.1139) -> (55.389, -147.0171)
  line L651 (55.389, -147.0171) -> (58.0178, -147.0171)
  line L652 (58.0178, -147.0171) -> (58.0178, -146.4467)
  line L653 (58.0178, -146.4468) -> (58.0197, -146.4372)
  line L654 (58.0197, -146.4372) -> (58.0333, -146.4237)
  line L655 (58.0333, -146.4237) -> (58.0428, -146.4218)
  line L656 (58.0428, -146.4218) -> (60.3991, -146.4218)
  line L657 (60.3991, -146.4218) -> (60.3991, -144.6608)
  line L658 (60.3991, -144.6608) -> (60.401, -144.6512)
  line L659 (60.401, -144.6512) -> (60.4145, -144.6377)
  line L660 (60.4145, -144.6377) -> (60.4241, -144.6358)
  line L661 (60.4241, -144.6358) -> (61.9124, -144.6358)
  line L662 (61.9124, -144.6358) -> (61.9219, -144.6377)
  line L663 (61.9219, -144.6377) -> (61.9355, -144.6512)
  line L664 (61.9355, -144.6512) -> (61.9374, -144.6608)
  line L665 (61.9374, -144.6608) -> (61.9374, -147.6124)
  line L666 (61.9374, -147.6124) -> (62.21, -147.6124)
  line L667 (62.21, -147.6124) -> (66.6499, -147.6124)
  line L668 (66.6499, -147.6124) -> (66.6499, -146.4468)
  line L669 (66.6499, -146.4468) -> (66.6499, -142.5772)
  line L670 (66.6499, -142.5772) -> (66.6518, -142.5677)
  line L671 (66.6518, -142.5677) -> (66.6653, -142.5541)
  line L672 (66.6653, -142.5541) -> (66.6749, -142.5522)
  line L673 (66.6749, -142.5522) -> (69.3288, -142.5522)
  line L674 (69.3288, -142.5522) -> (69.3288, -141.6843)
  line L675 (69.3288, -141.6843) -> (69.3307, -141.6747)
  line L676 (69.3307, -141.6747) -> (69.3442, -141.6612)
  line L677 (69.3442, -141.6612) -> (69.3538, -141.6593)
  line L678 (69.3538, -141.6593) -> (71.71, -141.6593)
  line L679 (71.71, -141.6593) -> (71.71, -138.1374)
  line L680 (71.71, -138.1374) -> (67.8656, -138.1374)
  line L681 (67.8656, -138.1374) -> (67.856, -138.1355)
  line L682 (67.856, -138.1355) -> (67.8425, -138.122)
  line L683 (67.8425, -138.122) -> (67.8425, -138.122)
  line L684 (67.8425, -138.122) -> (67.8406, -138.1124)
  line L685 (67.8406, -138.1124) -> (67.8406, -136.9468)
  line L686 (67.8406, -136.9468) -> (60.7468, -136.9468)
  line L687 (73.2329, -143.7448) -> (73.2465, -143.7583)
  line L688 (73.2465, -143.7583) -> (73.2484, -143.7678)
  line L689 (73.2484, -143.7678) -> (73.2484, -146.7444)
  line L690 (73.2484, -146.7444) -> (73.2465, -146.754)
  line L691 (73.2465, -146.754) -> (73.2329, -146.7675)
  line L692 (73.2329, -146.7675) -> (73.2234, -146.7694)
  line L693 (73.2234, -146.7694) -> (69.3538, -146.7694)
  line L694 (69.3538, -146.7694) -> (69.1171, -146.7508)
  line L695 (69.1171, -146.7508) -> (68.8862, -146.6953)
  line L696 (68.8862, -146.6953) -> (68.6668, -146.6045)
  line L697 (68.6668, -146.6045) -> (68.4644, -146.4804)
  line L698 (68.4644, -146.4804) -> (68.2838, -146.3262)
  line L699 (68.2838, -146.3262) -> (68.1296, -146.1456)
  line L700 (68.1296, -146.1456) -> (68.0055, -145.9431)
  line L701 (68.0055, -145.9431) -> (67.9146, -145.7238)
  line L702 (67.9146, -145.7238) -> (67.8592, -145.4929)
  line L703 (67.8592, -145.4929) -> (67.8406, -145.2561)
  line L704 (67.8406, -145.2561) -> (67.8592, -145.0194)
  line L705 (67.8592, -145.0194) -> (67.9146, -144.7885)
  line L706 (67.9146, -144.7885) -> (68.0055, -144.5691)
  line L707 (68.0055, -144.5691) -> (68.1296, -144.3666)
  line L708 (68.1296, -144.3666) -> (68.2838, -144.1861)
  line L709 (68.2838, -144.1861) -> (68.4644, -144.0319)
  line L710 (68.4644, -144.0319) -> (68.6668, -143.9078)
  line L711 (68.6668, -143.9078) -> (68.8862, -143.8169)
  line L712 (68.8862, -143.8169) -> (69.1171, -143.7615)
  line L713 (69.1171, -143.7615) -> (69.3538, -143.7429)
  line L714 (69.3538, -143.7429) -> (69.3538, -143.7428)
  line L715 (69.3538, -143.7428) -> (73.2234, -143.7428)
  line L716 (73.2234, -143.7428) -> (73.2329, -143.7448)
  line L717 (69.3538, -143.7928) -> (69.3538, -143.7928)
  line L718 (69.3538, -143.7928) -> (69.2387, -143.7929)
  line L719 (69.2387, -143.7929) -> (69.0112, -143.8289)
  line L720 (69.0112, -143.8289) -> (68.7921, -143.9001)
  line L721 (68.7921, -143.9001) -> (68.5869, -144.0046)
  line L722 (68.5869, -144.0046) -> (68.4006, -144.14)
  line L723 (68.4006, -144.14) -> (68.2377, -144.3029)
  line L724 (68.2377, -144.3029) -> (68.1023, -144.4892)
  line L725 (68.1023, -144.4892) -> (67.9978, -144.6944)
  line L726 (67.9978, -144.6944) -> (67.9266, -144.9135)
  line L727 (67.9266, -144.9135) -> (67.8906, -145.141)
  line L728 (67.8906, -145.141) -> (67.8906, -145.3713)
  line L729 (67.8906, -145.3713) -> (67.9266, -145.5988)
  line L730 (67.9266, -145.5988) -> (67.9978, -145.8178)
  line L731 (67.9978, -145.8178) -> (68.1023, -146.0231)
  line L732 (68.1023, -146.0231) -> (68.2377, -146.2094)
  line L733 (68.2377, -146.2094) -> (68.4006, -146.3723)
  line L734 (68.4006, -146.3723) -> (68.5869, -146.5076)
  line L735 (68.5869, -146.5076) -> (68.7921, -146.6122)
  line L736 (68.7921, -146.6122) -> (69.0112, -146.6834)
  line L737 (69.0112, -146.6834) -> (69.2387, -146.7194)
  line L738 (69.2387, -146.7194) -> (69.3538, -146.7194)
  line L739 (69.3538, -146.7194) -> (73.1984, -146.7194)
  line L740 (73.1984, -146.7194) -> (73.1984, -143.7928)
  line L741 (73.1984, -143.7928) -> (69.3538, -143.7928)
  line L742 (143.0862, -141.9754) -> (143.2909, -142.0302)
  line L743 (143.2909, -142.0302) -> (143.4829, -142.1197)
  line L744 (143.4829, -142.1197) -> (143.6565, -142.2413)
  line L745 (143.6565, -142.2413) -> (143.8063, -142.3911)
  line L746 (143.8063, -142.3911) -> (143.9279, -142.5647)
  line L747 (143.9279, -142.5647) -> (144.0174, -142.7567)
  line L748 (144.0174, -142.7567) -> (144.0723, -142.9614)
  line L749 (144.0723, -142.9614) -> (144.0907, -143.1725)
  line L750 (144.0907, -143.1725) -> (144.0723, -143.3836)
  line L751 (144.0723, -143.3836) -> (144.0174, -143.5883)
  line L752 (144.0174, -143.5883) -> (143.9279, -143.7803)
  line L753 (143.9279, -143.7803) -> (143.8063, -143.9539)
  line L754 (143.8063, -143.9539) -> (143.6565, -144.1037)
  line L755 (143.6565, -144.1037) -> (143.4829, -144.2253)
  line L756 (143.4829, -144.2253) -> (143.2909, -144.3148)
  line L757 (143.2909, -144.3148) -> (143.0862, -144.3697)
  line L758 (143.0862, -144.3697) -> (142.8751, -144.3881)
  line L759 (142.8751, -144.3881) -> (142.664, -144.3697)
  line L760 (142.664, -144.3697) -> (142.4594, -144.3148)
  line L761 (142.4594, -144.3148) -> (142.2673, -144.2253)
  line L762 (142.2673, -144.2253) -> (142.0937, -144.1037)
  line L763 (142.0937, -144.1037) -> (141.9439, -143.9539)
  line L764 (141.9439, -143.9539) -> (141.8224, -143.7803)
  line L765 (141.8224, -143.7803) -> (141.7328, -143.5883)
  line L766 (141.7328, -143.5883) -> (141.678, -143.3836)
  line L767 (141.678, -143.3836) -> (141.6595, -143.1725)
  line L768 (141.6595, -143.1725) -> (141.678, -142.9614)
  line L769 (141.678, -142.9614) -> (141.7328, -142.7567)
  line L770 (141.7328, -142.7567) -> (141.8224, -142.5647)
  line L771 (141.8224, -142.5647) -> (141.9439, -142.3911)
  line L772 (141.9439, -142.3911) -> (142.0937, -142.2413)
  line L773 (142.0937, -142.2413) -> (142.2673, -142.1197)
  line L774 (142.2673, -142.1197) -> (142.4594, -142.0302)
  line L775 (142.4594, -142.0302) -> (142.664, -141.9754)
  line L776 (142.664, -141.9754) -> (142.8751, -141.9569)
  line L777 (142.8751, -141.9569) -> (143.0862, -141.9754)
  line L778 (141.7244, -143.3876) -> (141.7836, -143.5954)
  line L779 (141.7836, -143.5954) -> (141.8798, -143.7888)
  line L780 (141.8798, -143.7888) -> (142.01, -143.9611)
  line L781 (142.01, -143.9611) -> (142.1697, -144.1067)
  line L782 (142.1697, -144.1067) -> (142.3533, -144.2204)
  line L783 (142.3533, -144.2204) -> (142.5548, -144.2984)
  line L784 (142.5548, -144.2984) -> (142.7671, -144.3381)
  line L785 (142.7671, -144.3381) -> (142.9831, -144.3381)
  line L786 (142.9831, -144.3381) -> (143.1955, -144.2984)
  line L787 (143.1955, -144.2984) -> (143.3969, -144.2204)
  line L788 (143.3969, -144.2204) -> (143.5806, -144.1067)
  line L789 (143.5806, -144.1067) -> (143.7402, -143.9611)
  line L790 (143.7402, -143.9611) -> (143.8704, -143.7888)
  line L791 (143.8704, -143.7888) -> (143.9667, -143.5954)
  line L792 (143.9667, -143.5954) -> (144.0258, -143.3876)
  line L793 (144.0258, -143.3876) -> (144.0457, -143.1725)
  line L794 (144.0457, -143.1725) -> (144.0258, -142.9574)
  line L795 (144.0258, -142.9574) -> (143.9667, -142.7496)
  line L796 (143.9667, -142.7496) -> (143.8704, -142.5563)
  line L797 (143.8704, -142.5563) -> (143.7402, -142.3839)
  line L798 (143.7402, -142.3839) -> (143.5806, -142.2383)
  line L799 (143.5806, -142.2383) -> (143.3969, -142.1246)
  line L800 (143.3969, -142.1246) -> (143.1955, -142.0466)
  line L801 (143.1955, -142.0466) -> (142.9831, -142.0069)
  line L802 (142.9831, -142.0069) -> (142.7671, -142.0069)
  line L803 (142.7671, -142.0069) -> (142.5548, -142.0466)
  line L804 (142.5548, -142.0466) -> (142.3533, -142.1246)
  line L805 (142.3533, -142.1246) -> (142.1697, -142.2383)
  line L806 (142.1697, -142.2383) -> (142.01, -142.3839)
  line L807 (142.01, -142.3839) -> (141.8798, -142.5563)
  line L808 (141.8798, -142.5563) -> (141.7836, -142.7496)
  line L809 (141.7836, -142.7496) -> (141.7244, -142.9574)
  line L810 (141.7244, -142.9574) -> (141.7045, -143.1725)
  line L811 (141.7045, -143.1725) -> (141.7244, -143.3876)
  line L812 (138.8721, -135.3894) -> (138.8856, -135.4029)
  line L813 (138.8856, -135.4029) -> (138.8875, -135.4125)
  line L814 (138.8875, -135.4125) -> (138.8875, -140.8125)
  line L815 (138.8875, -140.8125) -> (138.8856, -140.8221)
  line L816 (138.8856, -140.8221) -> (138.8721, -140.8356)
  line L817 (138.8721, -140.8356) -> (138.8625, -140.8375)
  line L818 (138.8625, -140.8375) -> (137.3625, -140.8375)
  line L819 (137.3625, -140.8375) -> (137.3529, -140.8356)
  line L820 (137.3529, -140.8356) -> (137.3394, -140.8221)
  line L821 (137.3394, -140.8221) -> (137.3375, -140.8125)
  line L822 (137.3375, -140.8125) -> (137.3375, -135.4125)
  line L823 (137.3375, -135.4125) -> (137.3394, -135.4029)
  line L824 (137.3394, -135.4029) -> (137.3529, -135.3894)
  line L825 (137.3529, -135.3894) -> (137.3625, -135.3875)
  line L826 (137.3625, -135.3875) -> (138.8625, -135.3875)
  line L827 (138.8625, -135.3875) -> (138.8721, -135.3894)
  line L828 (137.3875, -135.4375) -> (137.3875, -140.7875)
  line L829 (137.3875, -140.7875) -> (138.8375, -140.7875)
  line L830 (138.8375, -140.7875) -> (138.8375, -135.4375)
  line L831 (138.8375, -135.4375) -> (137.3875, -135.4375)
  line L832 (88.4346, -132.5769) -> (88.4481, -132.5904)
  line L833 (88.4481, -132.5904) -> (88.45, -132.6)
  line L834 (88.45, -132.6) -> (88.45, -134.1)
  line L835 (88.45, -134.1) -> (88.4481, -134.1096)
  line L836 (88.4481, -134.1096) -> (88.4346, -134.1231)
  line L837 (88.4346, -134.1231) -> (88.425, -134.125)
  line L838 (88.425, -134.125) -> (83.025, -134.125)
  line L839 (83.025, -134.125) -> (83.0154, -134.1231)
  line L840 (83.0154, -134.1231) -> (83.0019, -134.1096)
  line L841 (83.0019, -134.1096) -> (83, -134.1)
  line L842 (83, -134.1) -> (83, -132.6)
  line L843 (83, -132.6) -> (83.0019, -132.5904)
  line L844 (83.0019, -132.5904) -> (83.0154, -132.5769)
  line L845 (83.0154, -132.5769) -> (83.025, -132.575)
  line L846 (83.025, -132.575) -> (88.425, -132.575)
  line L847 (88.425, -132.575) -> (88.4346, -132.5769)
  line L848 (83.05, -132.625) -> (83.05, -134.075)
  line L849 (83.05, -134.075) -> (88.4, -134.075)
  line L850 (88.4, -134.075) -> (88.4, -132.625)
  line L851 (88.4, -132.625) -> (83.05, -132.625)
  line L852 (107.4846, -132.5769) -> (107.4981, -132.5904)
  line L853 (107.4981, -132.5904) -> (107.5, -132.6)
  line L854 (107.5, -132.6) -> (107.5, -134.1)
  line L855 (107.5, -134.1) -> (107.4981, -134.1096)
  line L856 (107.4981, -134.1096) -> (107.4846, -134.1231)
  line L857 (107.4846, -134.1231) -> (107.475, -134.125)
  line L858 (107.475, -134.125) -> (102.075, -134.125)
  line L859 (102.075, -134.125) -> (102.0654, -134.1231)
  line L860 (102.0654, -134.1231) -> (102.0519, -134.1096)
  line L861 (102.0519, -134.1096) -> (102.05, -134.1)
  line L862 (102.05, -134.1) -> (102.05, -132.6)
  line L863 (102.05, -132.6) -> (102.0519, -132.5904)
  line L864 (102.0519, -132.5904) -> (102.0654, -132.5769)
  line L865 (102.0654, -132.5769) -> (102.075, -132.575)
  line L866 (102.075, -132.575) -> (107.475, -132.575)
  line L867 (107.475, -132.575) -> (107.4846, -132.5769)
  line L868 (102.1, -132.625) -> (102.1, -134.075)
  line L869 (102.1, -134.075) -> (107.45, -134.075)
  line L870 (107.45, -134.075) -> (107.45, -132.625)
  line L871 (107.45, -132.625) -> (102.1, -132.625)